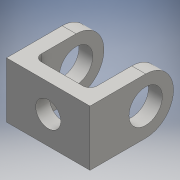
# Autodesk Inventor part: Damper_Mount_03
Saved by Autodesk Inventor 2016 (Build 200138000, 138)
## iProperties
Created: 2016-02-09
Part Number: Damper_Mount_03
Material: Generic
Document SubType Name: Modeling
Designer: nils
Density: 1 g/cm^3
Appearance: Default
Mass: 5.69253 g
Surface Area: 36.6661 cm^2
Volume: 5.69253 cm^3
Author: nils
Autodesk Inventor part; units mm, degrees
ref_plane "YZ Plane" through (0, 0, 0) normal (1, 0, 0) x (0, 1, 0)
ref_plane "XZ Plane" through (0, 0, 0) normal (0, 1, 0) x (-1, 0, 0)
ref_plane "XY Plane" through (0, 0, 0) normal (0, 0, 1) x (1, 0, 0)
sketch "Sketch1" plane through (0, 0, 0) normal (1, 0, 0) x (0, 1, 0)
  line L0 (0, 0) -> (30, 0)
  line L1 (30, 0) -> (30, -20)
  line L2 (30, -20) -> (0, -20)
  line L3 (0, -20) -> (0, 0)
  dimension "d0" = 30
  dimension "d1" = 20
  constraints: 8 end point, 2 parallel, 1 horizontal, 1 perpendicular
  measures "d0" distance of L1.end L2.end
  measures "d1" distance of L0.end L1.end
extrude "Extrusion1" add sketch "Sketch1" along normal blind 30
sketch "Sketch2" plane through (0, 30, 0) normal (0, 1, 0) x (1, 0, 0)
  line L0 (0, 0) -> (30, 0) projected
  line L1 (0, 20) -> (30, 20) projected
  line L2 (5, 0) -> (25, 0)
  line L3 (25, 0) -> (25, 20)
  line L4 (25, 20) -> (5, 20)
  line L5 (5, 20) -> (5, 0)
  line L6 (30, 20) -> (30, 0) projected
  dimension "d4" = 5
  dimension "d5" = 5
  constraints: 8 end point, 2 parallel, 2 point on line, 1 horizontal, 1 perpendicular
  measures "d4" distance from line of L5 L0.start
  measures "d5" distance from line of L6 L2.end
extrude "Extrusion2" cut sketch "Sketch2" against normal blind 25 contours L5 L1 L3 L0
fillet "Fillet1" radius 2.5 2 edges at (5, 5, -10) (25, 5, -10)
hole "Hole1" at (0, 20, -10) direction (1, 0, 0) diameter 12 end through all
fillet "Fillet3" radius 10 4 edges at (27.5, 30, -20) (2.5, 30, -20) (2.5, 30, 0) (27.5, 30, 0)
sketch "Sketch4" plane through (0, 5, 0) normal (0, 1, 0) x (1, 0, 0)
  line L0 (0, 4) -> (0, 16) projected
  line L1 (0, 10) -> (30, 10)
  line L2 (30, 20) -> (30, 0) projected
  point P0 (0, 0)
  point P1 (15, 10)
  constraints: 3 midpoint, 2 end point
hole "Hole2" at (15, 5, -10) direction (0, -1, 0) diameter 9 end through all
body "Solid1"
